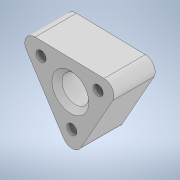
# Autodesk Inventor part: leg_fixer_1
Saved by Autodesk Inventor 2020 (Build 240168000, 168)
## iProperties
Created: 2020-08-19
Part Number: leg_fixer_1
Material: Generic
Document SubType Name: Modeling
Designer: psrobotics
Density: 1 g/cm^3
Appearance: Default
Author: psrobotics
Autodesk Inventor part; units mm, degrees
ref_plane "YZ Plane" through (0, 0, 0) normal (1, 0, 0) x (0, 1, 0)
ref_plane "XZ Plane" through (0, 0, 0) normal (0, 1, 0) x (-1, 0, 0)
ref_plane "XY Plane" through (0, 0, 0) normal (0, 0, 1) x (1, 0, 0)
sketch "Sketch1" plane through (0, 0, 0) normal (0, 0, 1) x (1, 0, 0)
  circle A0 centre (76.5892, -34.383) radius 2.05 projected
  circle A1 centre (85.7696, -48.6911) radius 2.05 projected
  circle A2 centre (93.5857, -34.7301) radius 2.05 projected
  line L0 (85.7696, -48.6911) -> (76.5892, -34.383) construction
  line L1 (88.2945, -47.071) -> (79.1142, -32.7629)
  line L2 (74.0643, -36.003) -> (83.2446, -50.3111)
  arc A3 (83.2446, -50.3111) -> (88.2945, -47.071) centre (85.7696, -48.6911) ccw
  arc A4 (79.1142, -32.7629) -> (74.0643, -36.003) centre (76.5892, -34.383) ccw
  line L3 (76.5892, -34.383) -> (93.5857, -34.7301) construction
  line L4 (76.528, -37.3823) -> (93.5244, -37.7295)
  line L5 (93.647, -31.7307) -> (76.6505, -31.3836)
  arc A5 (76.6505, -31.3836) -> (76.528, -37.3823) centre (76.5892, -34.383) ccw
  arc A6 (93.5244, -37.7295) -> (93.647, -31.7307) centre (93.5857, -34.7301) ccw
  line L6 (93.5857, -34.7301) -> (85.7696, -48.6911) construction
  line L7 (90.968, -33.2646) -> (83.1519, -47.2255)
  line L8 (88.3873, -50.1566) -> (96.2034, -36.1956)
  arc A7 (96.2034, -36.1956) -> (90.968, -33.2646) centre (93.5857, -34.7301) ccw
  arc A8 (83.1519, -47.2255) -> (88.3873, -50.1566) centre (85.7696, -48.6911) ccw
  circle A9 centre (85.7696, -48.6911) radius 1.5
  circle A10 centre (93.5857, -34.7301) radius 1.5
  circle A11 centre (76.5892, -34.383) radius 1.5
  point P0 (0, 0)
  point P1 (81.1794, -41.537)
  point P2 (85.0875, -34.5565)
  point P3 (89.6776, -41.7106)
  dimension "d0" = 6
  dimension "d1" = 6
  dimension "d2" = 6
  dimension "d3" = 3
  dimension "d4" = 3
  dimension "d5" = 3
  constraints: 24 end point, 12 point on circle, 12 tangent, 9 centre point, 3 coincident, 3 midpoint, 3 parallel
  measures "d0" diameter of A4
  measures "d1" diameter of A6
  measures "d2" diameter of A8
  measures "d3" diameter of A9
  measures "d4" diameter of A10
  measures "d5" diameter of A11
ref_plane "Work Plane1" through (82.5607, -52.1105, 12.3) normal (0, 0, 1) x (0.9725249, 0.2327991, 0)
extrude "Extrusion1" add sketch "Sketch1" along normal up to surface (12.3 mm away) contours A0 | A1 | A2 | A3 A8 L7 L1 | L1 L7 L4 A6 L8 A3 | L7 A8 L2 A5 L4 L1 | L1 L4 L7 | L4 A5 A4 L1 | L1 A4 L5 A7 L7 L4 | L7 A7 A6 L4
sketch "Sketch2" plane through (83.2446, -50.3111, 12.3) normal (0, 0, 1) x (0.8416525, 0.5400196, 0)
  circle A0 centre (3, 17) radius 1.5 projected
  circle A1 centre (3, 0) radius 1.5 projected
  circle A2 centre (17.1176, 7.5294) radius 1.5 projected
  arc A3 (4.6713, 19.4913) -> (0, 17) centre (3, 17) ccw projected
  line L0 (0, 0) -> (0, 17) projected
  arc A4 (0, 0) -> (4.4118, -2.6471) centre (3, 0) ccw projected
  line L1 (18.5294, 4.8824) -> (4.4118, -2.6471) projected
  arc A5 (18.5294, 4.8824) -> (18.7889, 10.0208) centre (17.1176, 7.5294) ccw projected
  line L2 (4.6713, 19.4913) -> (18.7889, 10.0208) projected
  line L3 (4.4118, -2.6471) -> (18.5294, 4.8824) projected
  line L4 (11.4706, 1.1176) -> (3, 17)
  line L5 (7.2353, 9.0588) -> (7.7059, 8.1765)
  circle A6 centre (7.7059, 8.1765) radius 4
  point P0 (-42.8941, 87.2982)
  dimension "d8" = 1
  dimension "d9" = 8
  constraints: 4 end point, 2 midpoint, 1 centre point, 1 coincident, 1 perpendicular, 1 point on line
  measures "d8" distance of L5.start L5.end
  measures "d9" diameter of A6
extrude "Extrusion2" cut sketch "Sketch2" against normal blind 14 contours L4 A6 | L4 A6
chamfer "Chamfer1" distance 1.5 angle 45 2 edges at (81.9482, -41.4281, 12.3) (81.9482, -41.4281, 0)
thicken "Thicken1" operation add thickness 1 both sides no extend neighbours yes toward (0.0204199, 0.9997915, 0) faces at (87.9815, -31.615, 4.1)
thicken "Thicken2" operation add thickness 1 both sides no extend neighbours yes toward (-0.8416525, -0.5400196, 0) faces at (76.6909, -40.0967, 4.1)
thicken "Thicken3" operation add thickness 1 both sides no extend neighbours yes toward (0.8725596, -0.4885077, 0) faces at (90.8081, -45.8326, 8.2)
body "Solid1"
